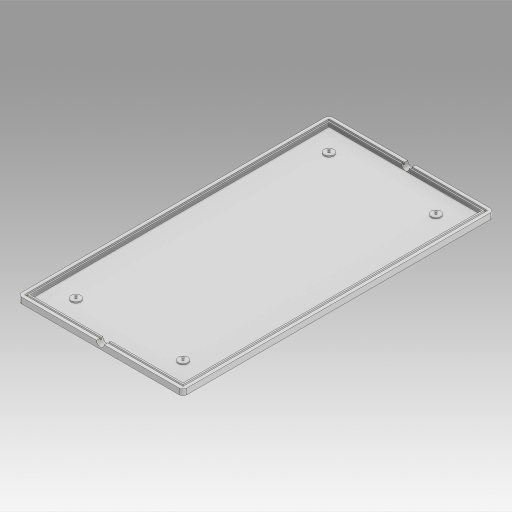
# Autodesk Inventor part: BOTTOM_COVER
Saved by Autodesk Inventor 2023 (Build 270158000, 158)
## iProperties
Created: 2025-09-17
Part Number: BOTTOM_COVER
Material: Generic
Document SubType Name: Modeling
Designer: NELLY NDUNG'U
Density: 1 g/cm^3
Appearance: Default
Author: NELLY NDUNG'U
Autodesk Inventor part; units mm, degrees
ref_plane "YZ Plane" through (0, 0, 0) normal (1, 0, 0) x (0, 1, 0)
ref_plane "XZ Plane" through (0, 0, 0) normal (0, 1, 0) x (-1, 0, 0)
ref_plane "XY Plane" through (0, 0, 0) normal (0, 0, 1) x (1, 0, 0)
sketch "Sketch1" plane through (0, 0, 0) normal (0, 1, 0) x (-1, 0, 0)
  line L0 (0, 0) -> (85, 0)
  line L1 (85, 0) -> (85, -160)
  line L2 (85, -160) -> (0, -160)
  line L3 (0, -160) -> (0, 0)
  dimension "d0" = 85
  dimension "d1" = 160
  constraints: 8 end point, 2 parallel, 1 horizontal, 1 perpendicular
  measures "d0" distance of L1.end L2.end
  measures "d1" distance of L0.end L1.end
extrude "Extrusion1" add sketch "Sketch1" along normal blind 3
fillet "Fillet1" radius 2 4 edges at (0, 1.5, 0) (-85, 1.5, 0) (-85, 1.5, -160) (0, 1.5, -160)
sketch "Sketch2" plane through (0, 3, 0) normal (0, 1, 0) x (1, 0, 0)
  arc A0 (0, 158) -> (-2, 160) centre (-2, 158) ccw projected
  line L0 (-2, 160) -> (-83, 160) projected
  arc A1 (-83, 160) -> (-85, 158) centre (-83, 158) ccw projected
  line L1 (-85, 158) -> (-85, 2) projected
  arc A2 (-85, 2) -> (-83, 0) centre (-83, 2) ccw projected
  line L2 (-83, 0) -> (-2, 0) projected
  arc A3 (-2, 0) -> (0, 2) centre (-2, 2) ccw projected
  line L3 (0, 2) -> (0, 158) projected
  line L4 (-82.5, 2.5) -> (-82.5, 157.5)
  line L5 (-82.5, 157.5) -> (-2.5, 157.5)
  line L6 (-2.5, 157.5) -> (-2.5, 2.5)
  line L7 (-2.5, 2.5) -> (-82.5, 2.5)
  line L8 (-81.75, 156.75) -> (-81.75, 3.25)
  line L9 (-81.75, 3.25) -> (-3.25, 3.25)
  line L10 (-3.25, 3.25) -> (-3.25, 156.75)
  line L11 (-3.25, 156.75) -> (-81.75, 156.75)
  line L12 (-83.25, 158.25) -> (-83.25, 1.75)
  line L13 (-83.25, 1.75) -> (-1.75, 1.75)
  line L14 (-1.75, 1.75) -> (-1.75, 158.25)
  line L15 (-1.75, 158.25) -> (-83.25, 158.25)
  point P0 (0, 0)
  dimension "d5" = 2.5
  dimension "d6" = 0.75
  dimension "d31" = 0.75
  constraints: 24 end point, 9 other
  measures "d5" distance between parallel lines of L1 L4
  measures "d6" distance between parallel lines of L4 L8
  measures "d31" distance between parallel lines of L4 L12
extrude "Extrusion2" cut sketch "Sketch2" against normal blind 2 contours L11 L10 L9 L8
extrude "Extrusion3" cut sketch "Sketch2" against normal blind 0.75 contours L15 L14 L13 L12
sketch "Sketch3" plane through (0, 1, 0) normal (0, 1, 0) x (1, 0, 0)
  circle A0 centre (-70, 15) radius 2.5
  circle A1 centre (-15, 15) radius 2.5
  circle A2 centre (-70, 145) radius 2.5
  circle A3 centre (-15, 145) radius 2.5
  circle A4 centre (-70, 15) radius 0.5
  circle A5 centre (-15, 15) radius 0.5
  circle A6 centre (-15, 145) radius 0.5
  circle A7 centre (-70, 145) radius 0.5
  line L0 (-85, 158) -> (-85, 2) projected
  line L1 (-83, 0) -> (-2, 0) projected
  line L2 (0, 2) -> (0, 158) projected
  line L3 (-2, 160) -> (-83, 160) projected
  point P0 (0, 0)
  dimension "d11" = 5
  dimension "d12" = 5
  dimension "d13" = 5
  dimension "d14" = 5
  dimension "d15" = 2
  dimension "d16" = 2
  dimension "d17" = 2
  dimension "d18" = 2
  dimension "d19" = 15
  dimension "d20" = 15
  dimension "d21" = 15
  dimension "d22" = 15
  dimension "d23" = 15
  dimension "d24" = 15
  dimension "d25" = 15
  dimension "d26" = 15
  constraints: 8 centre point
  measures "d11" diameter of A0
  measures "d12" diameter of A1
  measures "d13" diameter of A2
  measures "d14" diameter of A3
  measures "d15" radial gap between concentric circles of A0 A4
  measures "d16" radial gap between concentric circles of A1 A5
  measures "d17" radial gap between concentric circles of A3 A6
  measures "d18" radial gap between concentric circles of A2 A7
  measures "d19" distance from line of A0.centre L0
  measures "d20" distance from line of A0.centre L1
  measures "d21" distance from line of A1.centre L1
  measures "d22" distance from line of L2 A1.centre
  measures "d23" distance from line of L3 A3.centre
  measures "d24" distance from line of L2 A3.centre
  measures "d25" distance from line of L3 A2.centre
  measures "d26" distance from line of A2.centre L0
extrude "Extrusion4" add sketch "Sketch3" along normal blind 1.5 contours A4 | A5 | A6 | A7
extrude "Extrusion5" add sketch "Sketch3" along normal blind 0.5 contours A0 | A1 | A2 | A3 | A4 | A6
sketch "Sketch4" plane through (-2, 0, -160) normal (0, 0, -1) x (-1, 0, 0)
  line L0 (1.25, 3) -> (79.75, 3) projected
  arc A0 (38.5, 3) -> (42.5, 3) centre (40.5, 3) ccw
  line L1 (0, 0) -> (81, 0) projected
  line L2 (0, 3) -> (81, 3) projected
  line L3 (79.75, 1) -> (1.25, 1) projected
  point P0 (-2, 0)
  point P1 (-2, 3)
  point P2 (40.5, 3)
  point P3 (38.5, 3)
  dimension "d32" = 42.5
  dimension "d33" = 3
  constraints: 2 midpoint, 2 point on circle, 2 point on line, 1 centre point, 1 tangent
  measures "d32" distance of point (-2, 3) A0.centre
  measures "d33" distance from line of L1 point (40.5, 3)
extrude "Extrusion6" cut sketch "Sketch4" against normal through all
body "Solid1"
